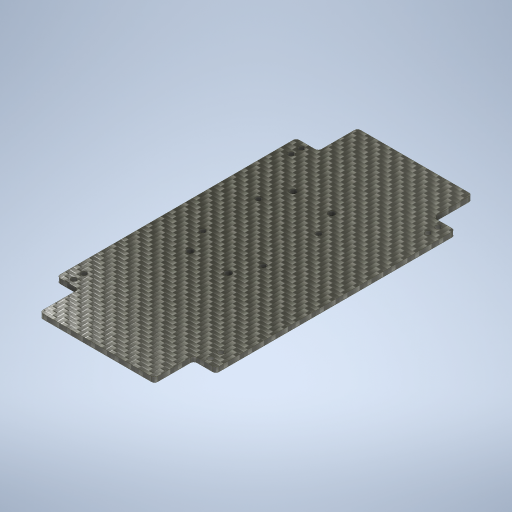
# Autodesk Inventor part: FootSoleFrame
Saved by Autodesk Inventor 2024.2 (Build 282272000, 272)
## iProperties
Created: 2024-01-07
Part Number: FootSoleFrame
Material: CFRP
Document SubType Name: Modeling
Designer: Masato Kubotera
Density: 1.43 g/cm^3
Appearance: Carbon Fiber 1
Mass: 79.1828 g
Surface Area: 392.308 cm^2
Volume: 55.3726 cm^3
Vendor: ALLPCB
Author: Masato Kubotera
Autodesk Inventor part; units mm, degrees
ref_plane "YZ Plane" through (0, 0, 0) normal (1, 0, 0) x (0, 1, 0)
ref_plane "XZ Plane" through (0, 0, 0) normal (0, 1, 0) x (-1, 0, 0)
ref_plane "XY Plane" through (0, 0, 0) normal (0, 0, 1) x (1, 0, 0)
sketch "Sketch1" plane through (0, 0, 0) normal (0, 0, 1) x (1, 0, 0)
  line L0 (-100, 59.95) -> (100, 59.95)
  line L1 (100, 59.95) -> (100, -40.05)
  line L2 (100, -40.05) -> (-100, -40.05)
  line L3 (-100, -40.05) -> (-100, 59.95)
  line L4 (-100, 59.95) -> (100, -40.05) construction
  line L5 (100, 59.95) -> (-100, -40.05) construction
  line L6 (0, -40.05) -> (0, 59.95) construction
  line L7 (-100, 9.95) -> (100, 9.95) construction
  line L8 (-100, 0) -> (100, 0) construction
  line L9 (-44, -22.5) -> (18, -22.5) construction
  line L10 (18, -22.5) -> (18, 22.5) construction
  line L11 (18, 22.5) -> (-44, 22.5) construction
  line L12 (-44, 22.5) -> (-44, -22.5) construction
  line L13 (-44, -22.5) -> (18, 22.5) construction
  line L14 (18, -22.5) -> (-44, 22.5) construction
  line L15 (13, -22.5) -> (13, 22.5) construction
  line L16 (4.5, -19) -> (4.5, 19) construction
  line L17 (-13, -22.5) -> (-13, 22.5) construction
  line L18 (-39, -22.5) -> (-39, 22.5) construction
  line L19 (100, 46.05) -> (75.3, 46.05)
  line L20 (75.3, 46.05) -> (75.3, 59.95)
  line L21 (65.2, 49.05) -> (97, 49.05) construction
  line L22 (97, 49.05) -> (97, 56.95) construction
  line L23 (97, 56.95) -> (65.2, 56.95) construction
  line L24 (65.2, 56.95) -> (65.2, 49.05) construction
  line L25 (65.2, 49.05) -> (97, 56.95) construction
  line L26 (97, 49.05) -> (65.2, 56.95) construction
  line L27 (65.2, 53) -> (97, 53) construction
  line L28 (81.1, 49.05) -> (81.1, 56.95) construction
  circle A0 centre (71.55, 53) radius 1.75 construction
  circle A1 centre (65.2, 53) radius 1.75 construction
  line L29 (100, -26.15) -> (75.3, -26.15)
  line L30 (75.3, -26.15) -> (75.3, -40.05)
  line L31 (-100, 46.05) -> (-75.3, 46.05)
  line L32 (-75.3, 46.05) -> (-75.3, 59.95)
  line L33 (-75.3, -26.15) -> (-75.3, -40.05)
  line L34 (-100, -26.15) -> (-75.3, -26.15)
  line L35 (13, -12) -> (18, -12) construction
  line L36 (13, 12) -> (18, 12) construction
  point P0 (0, 0)
  point P1 (0, 9.95)
  point P2 (-13, 0)
  point P3 (-30.5, -19)
  point P4 (-30.5, 19)
  point P5 (81.1, 53)
  point P6 (90.65, 53)
  point P7 (-75.3, 59.95)
  point P8 (-75.3, -40.05)
  point P9 (75.3, -40.05)
  point P10 (65.2, -33.1)
  point P11 (71.55, -33.1)
  point P12 (-65.2, 53)
  point P13 (-71.55, 53)
  point P14 (-65.2, -33.1)
  point P15 (-71.55, -33.1)
  point P16 (19.5, -12)
  point P17 (19.5, 12)
  point P18 (-45.5, -12)
  point P19 (-45.5, 12)
  dimension "d0" = 200
  dimension "d1" = 100
  dimension "d2" = 62
  dimension "d3" = 45
  dimension "d4" = 80.1
  dimension "d5" = 5
  dimension "d7" = 38
  dimension "d8" = 35
  dimension "d9" = 31.8
  dimension "d10" = 7.9
  dimension "d11" = 19.1
  dimension "d12" = 3
  dimension "d13" = 3
  dimension "d14" = 3.5
  dimension "d15" = 2
  dimension "d27" = 87
  dimension "d28" = 24
  dimension "d29" = 1.5
  dimension "d37" = 6.95
  dimension "d38" = 4.5
  constraints: 74 end point, 24 symmetric about line, 17 midpoint, 15 point on line, 7 horizontal, 6 parallel, 5 coincident, 3 perpendicular, 3 vertical, 2 centre point, 1 equal radius, 2 other
  measures "d0" distance of L1.end L2.end
  measures "d1" distance of L0.end L1.end
  measures "d2" distance of L11.end L10.end
  measures "d3" distance of L10.end L9.end
  measures "d4" diameter of L2 L8
  measures "d5" distance between parallel lines of L10 L15
  measures "d7" distance of L16.end L16.start
  measures "d8" distance of point (4.5, 19) point (-30.5, 19)
  measures "d9" distance of L23.end L22.end
  measures "d10" distance of L22.end L21.end
  measures "d11" distance of point (71.55, 53) point (90.65, 53)
  measures "d12" distance between parallel lines of L0 L23
  measures "d13" distance between parallel lines of L1 L22
  measures "d14" diameter of A0
  measures "d15" distance edge to line of A0 L20
  measures "d27" distance between parallel lines of L3 L17
  measures "d28" distance between parallel lines of L36 L35
  measures "d29" distance from line of point (19.5, 12) L10
  measures "d37" distance between parallel lines of L0 L27
  measures "d38" distance between parallel lines of L16 L6
extrude "Extrusion1" add sketch "Sketch1" against normal blind 3 contours L0 L20 L19 L1 L29 L30 L2 L33 L34 L3 L31 L32
hole "Hole1" at (4.5, -19, 0) at (4.5, 19, 0) at (-30.5, -19, 0) at (-30.5, 19, 0) at (65.2, 53, 0) at (71.55, 53, 0) at (90.65, 53, 0) at (65.2, -33.1, 0) at (71.55, -33.1, 0) at (-71.55, -33.1, 0) at (-65.2, -33.1, 0) at (-65.2, 53, 0) at (-71.55, 53, 0) direction (0, 0, -1) diameter 3.5 end through all
fillet "Fillet1" radius 2 12 edges at (100, 46.05, -1.5) (100, -26.15, -1.5) (75.3, -40.05, -1.5) (75.3, -26.15, -1.5) (75.3, 46.05, -1.5) (75.3, 59.95, -1.5) (-75.3, 59.95, -1.5) (-75.3, 46.05, -1.5) (-100, 46.05, -1.5) (-100, -26.15, -1.5) (-75.3, -26.15, -1.5) (-75.3, -40.05, -1.5)
hole "Hole2" at (19.5, -12, 0) at (19.5, 12, 0) at (-45.5, -12, 0) at (-45.5, 12, 0) direction (0, 0, -1) diameter 4 end through all
equation "\"d13\" = d12"
equation "\"d19\" = d14"
body "Solid1"
